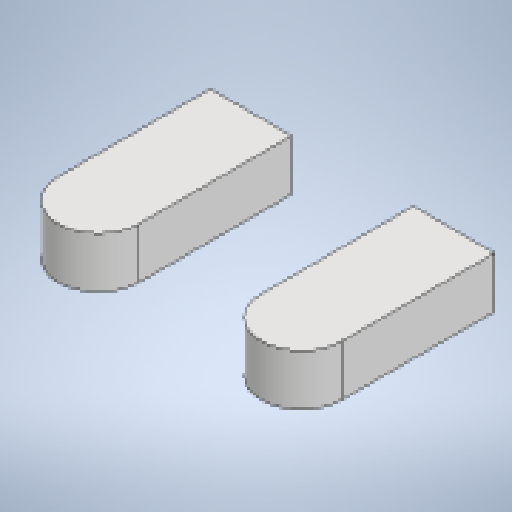
# Autodesk Inventor part: pallet jack dummy
Saved by Autodesk Inventor 2025.3 (Build 293356030, 356C)
## iProperties
Created: 2025-12-18
Part Number: pallet jack dummy
Material: Generic
Document SubType Name: Modeling
Designer: admin
Density: 1 g/cm^3
Appearance: Default
Author: admin
Autodesk Inventor part; units mm, degrees
ref_plane "YZ Plane" through (0, 0, 0) normal (1, 0, 0) x (0, 1, 0)
ref_plane "XZ Plane" through (0, 0, 0) normal (0, 1, 0) x (-1, 0, 0)
ref_plane "XY Plane" through (0, 0, 0) normal (0, 0, 1) x (1, 0, 0)
sketch "Sketch1" plane through (0, 0, 0) normal (0, 0, 1) x (1, 0, 0)
  line L0 (280, 0) -> (280, -300)
  arc A0 (120, -300) -> (280, -300) centre (200, -300) ccw
  line L1 (120, -300) -> (120, 0)
  line L2 (-120, 0) -> (-120, -300)
  arc A1 (-280, -300) -> (-120, -300) centre (-200, -300) ccw
  line L3 (-280, -300) -> (-280, 0)
  line L4 (280, 0) -> (-280, 0)
  line L5 (0, 0) -> (0, -525.5319) construction
  dimension "d0" = 160
  dimension "d1" = 560
  dimension "d2" = 300
  constraints: 12 end point, 4 point on circle, 4 tangent, 3 vertical, 2 centre point, 2 parallel, 1 equal radius, 1 horizontal, 1 midpoint, 1 point on line, 1 other
  measures "d0" distance between parallel lines of L1 L0
  measures "d1" distance between parallel lines of L3 L0
  measures "d2" distance from line of L4 A1.centre
extrude "Extrusion1" add sketch "Sketch1" along normal blind 100
body "Solid1"
